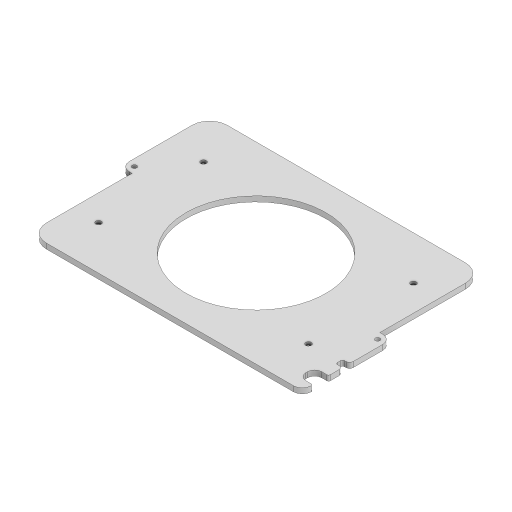
# Autodesk Inventor part: Microscope lid
Saved by Autodesk Inventor 2023 (Build 270158000, 158)
## iProperties
Created: 2022-05-13
Part Number: Microscope lid
Material: Generic
Document SubType Name: Modeling
Designer: ferrerx
Density: 1 g/cm^3
Appearance: Default
Author: ferrerx
Autodesk Inventor part; units mm, degrees
ref_plane "YZ Plane" through (0, 0, 0) normal (1, 0, 0) x (0, 1, 0)
ref_plane "XZ Plane" through (0, 0, 0) normal (0, 1, 0) x (-1, 0, 0)
ref_plane "XY Plane" through (0, 0, 0) normal (0, 0, 1) x (1, 0, 0)
sketch "Sketch1" plane through (0, 0, 0) normal (0, 1, 0) x (-1, 0, 0)
  circle A0 centre (0, 0) radius 40
  circle A1 centre (0, 0) radius 25
  dimension "d1" = 50
  dimension "d13" = 15
  constraints: 2 centre point, 2 coincident
  measures "d1" diameter of A1
  measures "d13" radial gap between concentric circles of A0 A1
extrude "Extrusion1" add sketch "Sketch1" along normal blind 5
sketch "Sketch2" plane through (0, 5, 0) normal (0, 1, 0) x (1, 0, 0)
  circle A0 centre (-33, 0) radius 1.25
  circle A1 centre (0, 0) radius 25 projected
  circle A2 centre (0, 0) radius 33 construction
  dimension "d4" = 2.5
  dimension "d12" = 8
  constraints: 1 centre point, 1 coincident, 1 horizontal alignment, 2 other
  measures "d4" diameter of A0
extrude "Extrusion2" cut sketch "Sketch2" against normal blind 10 contours A0
pattern_circular "Circular Pattern1" count 6 over 360 about axis through (0, 0, 0) along (0, 1, 0) of "Extrusion2"
sketch "Sketch3" plane through (0, 5, 0) normal (0, 1, 0) x (1, 0, 0)
  line L0 (-85, -42.5) -> (85, -42.5)
  line L1 (85, -42.5) -> (85, 42.5)
  line L2 (85, 42.5) -> (-85, 42.5)
  line L3 (-85, 42.5) -> (-85, -42.5)
  line L4 (-85, -42.5) -> (85, 42.5) construction
  line L5 (85, -42.5) -> (-85, 42.5) construction
  line L6 (34.5, 15.5) -> (65.5, 15.5) construction
  line L7 (65.5, 15.5) -> (65.5, -15.5) construction
  line L8 (65.5, -15.5) -> (34.5, -15.5) construction
  line L9 (34.5, -15.5) -> (34.5, 15.5) construction
  line L10 (34.5, 15.5) -> (65.5, -15.5) construction
  line L11 (65.5, 15.5) -> (34.5, -15.5) construction
  circle A0 centre (34.5, 15.5) radius 1.5
  circle A1 centre (65.5, 15.5) radius 1.5
  circle A2 centre (65.5, -15.5) radius 1.5
  circle A3 centre (34.5, -15.5) radius 1.5
  line L12 (0, 0) -> (50, 0) construction
  circle A4 centre (0, 0) radius 40
  circle A5 centre (0, 0) radius 40 projected
  line L13 (-50, 42.5) -> (-50, -42.5)
  circle A6 centre (50, 0) radius 12
  dimension "d14" = 85
  dimension "d15" = 170
  dimension "d16" = 31
  dimension "d17" = 31
  dimension "d18" = 3
  dimension "d19" = 3
  dimension "d20" = 3
  dimension "d21" = 3
  dimension "d22" = 50
  dimension "d23" = 35
  dimension "d26" = 24
  constraints: 28 end point, 6 centre point, 6 coincident, 4 midpoint, 4 parallel, 3 horizontal, 3 perpendicular, 2 point on line, 1 concentric
  measures "d14" distance of L0.end L1.end
  measures "d15" distance of L0.start L0.end
  measures "d16" distance of L6.start L6.end
  measures "d17" distance of L8.end L6.start
  measures "d18" diameter of A1
  measures "d19" diameter of A0
  measures "d20" diameter of A3
  measures "d21" diameter of A2
  measures "d22" distance of L12.start L12.end
  measures "d23" distance between parallel lines of L3 L13
  measures "d26" diameter of A6
extrude "Extrusion3" add sketch "Sketch3" against normal blind 5 contours L13 L2 L1 L0
sketch "Sketch4" plane through (0, 5, 0) normal (0, 1, 0) x (1, 0, 0)
  arc A0 (39.56, -5.9166) -> (39.56, 5.9166) centre (50, 0) ccw projected
  circle A1 centre (50, 0) radius 12
  point P0 (0, 0)
  point P1 (39.56, 5.9166)
  point P2 (39.56, -5.9166)
  constraints: 1 centre point, 1 coincident
extrude "Extrusion4" cut sketch "Sketch4" against normal blind 5
sketch "Sketch5" plane through (0, 5, 0) normal (0, 1, 0) x (1, 0, 0)
  circle A0 centre (65.5, 15.5) radius 1.5 projected
  circle A1 centre (65.5, 15.5) radius 1.5
  line L0 (34.5, -15.5) -> (65.5, -15.5)
  line L1 (65.5, -15.5) -> (65.5, 15.5)
  line L2 (65.5, 15.5) -> (34.5, 15.5)
  line L3 (34.5, 15.5) -> (34.5, -15.5)
  circle A2 centre (50, 0) radius 12 projected
  line L4 (34.5, -15.5) -> (65.5, 15.5) construction
  line L5 (65.5, -15.5) -> (34.5, 15.5) construction
  circle A3 centre (34.5, 15.5) radius 1.5
  circle A4 centre (34.5, -15.5) radius 1.5
  point P0 (0, 0)
  dimension "d30" = 3
  dimension "d31" = 3
  constraints: 12 end point, 3 centre point, 3 coincident, 2 midpoint, 2 parallel, 1 horizontal, 1 perpendicular
  measures "d30" diameter of A3
  measures "d31" diameter of A4
extrude "Extrusion5" cut sketch "Sketch5" against normal blind 5 contours A3 L3 L2 | L2 L3 A3 | A4 L3 L0 | L0 L3 A4
sketch "Sketch6" plane through (0, 5, 0) normal (0, 1, 0) x (1, 0, 0)
  line L0 (-65.5, -55) -> (97.5, -55)
  line L1 (97.5, -55) -> (97.5, 55)
  line L2 (97.5, 55) -> (-65.5, 55)
  line L3 (-65.5, 55) -> (-65.5, -55)
  line L4 (-65.5, -55) -> (97.5, 55) construction
  line L5 (97.5, -55) -> (-65.5, 55) construction
  line L6 (-65.5, 4) -> (-58.8, 4)
  line L7 (-58.8, 4) -> (-58.8, -55)
  line L8 (-58.8, -55) -> (-65.5, -55)
  line L9 (-65.5, -55) -> (-65.5, 4)
  line L10 (97.5, 55) -> (90.8, 55)
  line L11 (90.8, 55) -> (90.8, -4)
  line L12 (90.8, -4) -> (97.5, -4)
  line L13 (97.5, -4) -> (97.5, 55)
  line L14 (-50, -42.5) -> (-50, 42.5) projected
  line L15 (85, 42.5) -> (85, -42.5) projected
  line L16 (-50, 42.5) -> (85, 42.5)
  line L17 (85, 42.5) -> (85, -42.5)
  line L18 (85, -42.5) -> (-50, -42.5)
  line L19 (-50, -42.5) -> (-50, 42.5)
  point P0 (0, 0)
  point P1 (16, 0)
  dimension "d34" = 16
  dimension "d35" = 110
  dimension "d36" = 163
  dimension "d37" = 6.7
  dimension "d38" = 6.7
  dimension "d40" = 51
  dimension "d41" = 51
  constraints: 36 end point, 8 parallel, 4 horizontal, 4 perpendicular, 2 midpoint, 2 point on line
  measures "d34" distance of point (0, 0) point (16, 0)
  measures "d35" distance of L0.end L1.end
  measures "d36" distance of L0.start L0.end
  measures "d37" distance between parallel lines of L1 L11
  measures "d38" distance between parallel lines of L3 L7
  measures "d40" distance between parallel lines of L2 L6
  measures "d41" distance between parallel lines of L0 L12
extrude "Extrusion6" add sketch "Sketch6" against normal blind 5 contours L7 L6 L3 L2 L11 L12 L1 L0
sketch "Sketch7" plane through (0, 5, 0) normal (0, 1, 0) x (1, 0, 0)
  line L0 (97.5, -49) -> (89.5, -49)
  line L1 (89.5, -49) -> (89.5, -40)
  line L2 (89.5, -40) -> (97.5, -40)
  line L3 (97.5, -40) -> (97.5, -49)
  line L4 (-58.8, -55) -> (97.5, -55) projected
  line L5 (97.5, -55) -> (97.5, -4) projected
  line L6 (97.5, -28) -> (93.5, -28)
  line L7 (93.5, -28) -> (93.5, -32)
  line L8 (93.5, -32) -> (97.5, -32)
  line L9 (97.5, -32) -> (97.5, -28)
  point P0 (0, 0)
  dimension "d44" = 6
  dimension "d45" = 9
  dimension "d46" = 8
  dimension "d47" = 8
  dimension "d48" = 4
  dimension "d49" = 4
  constraints: 16 end point, 4 parallel, 2 horizontal, 2 perpendicular, 1 collinear, 1 point on line
  measures "d44" distance between parallel lines of L4 L0
  measures "d45" distance of L0.end L1.end
  measures "d46" distance of L1.end L2.end
  measures "d47" distance between parallel lines of L2 L8
  measures "d48" distance of L6.end L7.end
  measures "d49" distance of L6.start L6.end
extrude "Extrusion7" cut sketch "Sketch7" against normal blind 5
fillet "Fillet2" radius 2 2 edges at (97.5, 2.5, 28) (97.5, 2.5, 32)
fillet "Fillet3" radius 1 2 edges at (93.5, 2.5, 28) (93.5, 2.5, 32)
fillet "Fillet4" radius 1 2 edges at (97.5, 2.5, 49) (97.5, 2.5, 40)
fillet "Fillet5" radius 5 1 edges at (97.5, 2.5, 55)
fillet "Fillet6" radius 4 2 edges at (89.5, 2.5, 40) (89.5, 2.5, 49)
fillet "Fillet7" radius 5 2 edges at (97.5, 2.5, 4) (-65.5, 2.5, -4)
fillet "Fillet8" radius 10 3 edges at (-58.8, 2.5, 55) (90.8, 2.5, -55) (-65.5, 2.5, -55)
sketch "Sketch8" plane through (0, 5, 0) normal (0, 1, 0) x (1, 0, 0)
  circle A0 centre (-61.5, 8) radius 1.35
  circle A1 centre (93.5, -8) radius 1.35
  line L0 (-60.5, 4) -> (-58.8, 4) projected
  line L1 (-65.5, 45) -> (-65.5, 9) projected
  line L2 (92.5, -4) -> (90.8, -4) projected
  line L3 (97.5, -26) -> (97.5, -9) projected
  point P0 (0, 0)
  dimension "d59" = 4
  dimension "d60" = 4
  dimension "d61" = 2.7
  dimension "d62" = 4
  dimension "d63" = 4
  dimension "d64" = 2.7
  constraints: 2 centre point
  measures "d59" distance from line of A0.centre L0
  measures "d60" distance from line of L1 A0.centre
  measures "d61" diameter of A0
  measures "d62" distance from line of L2 A1.centre
  measures "d63" distance from line of L3 A1.centre
  measures "d64" diameter of A1
extrude "Extrusion8" cut sketch "Sketch8" against normal blind 5
sketch "Sketch9" plane through (0, 5, 0) normal (0, 1, 0) x (1, 0, 0)
  line L0 (-48, 44) -> (76, 44)
  line L1 (76, 44) -> (76, -39)
  line L2 (76, -39) -> (-48, -39)
  line L3 (-48, -39) -> (-48, 44)
  point P0 (0, 0)
  constraints: 8 end point, 2 parallel, 1 horizontal, 1 perpendicular
extrude "Extrusion9" add sketch "Sketch9" against normal blind 5
sketch "Sketch10" plane through (0, 5, 0) normal (0, 1, 0) x (1, 0, 0)
  circle A0 centre (16, 0) radius 40
  line L0 (-58.8, 4) -> (-58.8, -45) projected
  point P0 (0, 0)
  dimension "d69" = 80
  dimension "d70" = 74.8
  constraints: 1 centre point
  measures "d69" diameter of A0
  measures "d70" distance from line of L0 A0.centre
extrude "Extrusion10" cut sketch "Sketch10" against normal blind 5
sketch "Sketch11" plane through (0, 5, 0) normal (0, 1, 0) x (1, 0, 0)
  line L0 (-44, -30) -> (76, -30) construction
  line L1 (76, -30) -> (76, 30) construction
  line L2 (76, 30) -> (-44, 30) construction
  line L3 (-44, 30) -> (-44, -30) construction
  circle A0 centre (16, 0) radius 40 construction
  line L4 (-44, -30) -> (76, 30) construction
  line L5 (76, -30) -> (-44, 30) construction
  circle A1 centre (76, 30) radius 1.6
  circle A2 centre (-44, 30) radius 1.6
  circle A3 centre (-44, -30) radius 1.6
  circle A4 centre (76, -30) radius 1.6
  point P0 (0, 0)
  dimension "d73" = 60
  dimension "d74" = 120
  dimension "d75" = 3.2
  dimension "d76" = 3.2
  dimension "d77" = 3.2
  dimension "d78" = 3.2
  constraints: 12 end point, 4 centre point, 4 coincident, 2 midpoint, 2 parallel, 1 horizontal, 1 perpendicular
  measures "d73" distance of L0.end L1.end
  measures "d74" distance of L0.start L0.end
  measures "d75" diameter of A4
  measures "d76" diameter of A1
  measures "d77" diameter of A2
  measures "d78" diameter of A3
extrude "Extrusion11" cut sketch "Sketch11" against normal blind 5
sketch "Sketch12" plane through (0, 5, 0) normal (0, 1, 0) x (1, 0, 0)
  line L0 (-160, 70) -> (160, 70)
  line L1 (160, 70) -> (160, -70)
  line L2 (160, -70) -> (-160, -70)
  line L3 (-160, -70) -> (-160, 70)
  line L4 (-160, 70) -> (160, -70) construction
  line L5 (160, 70) -> (-160, -70) construction
  point P0 (0, 0)
  constraints: 12 end point, 2 midpoint, 2 parallel, 1 horizontal, 1 perpendicular
extrude "Extrusion12" cut sketch "Sketch12" against normal blind 2
chamfer "Chamfer1" distance 1.6 angle 45 4 edges at (-45.6, 0, 30) (74.4, 0, 30) (74.4, 0, -30) (-45.6, 0, -30)
body "Solid1"
